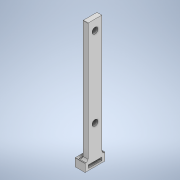
# Autodesk Inventor part: baseB
Saved by Autodesk Inventor 2021.4 (Build 254397000, 397)
## iProperties
Created: 2023-11-06
Part Number: baseB
Material: 一般
Document SubType Name: Modeling
Designer: ryusei
Density: 1 g/cm^3
Appearance: 既定
Author: ryusei
Autodesk Inventor part; units mm, degrees
ref_plane "YZ Plane" through (0, 0, 0) normal (1, 0, 0) x (0, 1, 0)
ref_plane "XZ Plane" through (0, 0, 0) normal (0, 1, 0) x (-1, 0, 0)
ref_plane "XY Plane" through (0, 0, 0) normal (0, 0, 1) x (1, 0, 0)
sketch "スケッチ1" plane through (0, 0, 0) normal (0, 1, 0) x (-1, 0, 0)
  line L0 (5, -10) -> (-5, -10)
  line L1 (-5, -10) -> (-5, 10)
  line L2 (-5, 10) -> (5, 10)
  line L3 (5, 10) -> (5, -10)
  line L4 (5, -10) -> (-5, 10) construction
  line L5 (-5, -10) -> (5, 10) construction
  point P0 (0, 0)
  dimension "d0" = 10
  dimension "d1" = 20
  constraints: 12 end point, 2 midpoint, 2 parallel, 1 horizontal, 1 perpendicular
  measures "d0" distance of L1.end L2.end
  measures "d1" distance of L0.end L1.end
extrude "押し出し1" add sketch "スケッチ1" along normal blind 6
sketch "スケッチ2" plane through (0, 0, 0) normal (0, -1, 0) x (1, 0, 0)
  line L0 (5, 10) -> (5, -10) projected
  circle A0 centre (5, 0) radius 6.75
  point P0 (0, 0)
  point P1 (5, -6.75)
  point P2 (5, 6.75)
  dimension "d4" = 13.5
  constraints: 1 centre point, 1 midpoint
  measures "d4" diameter of A0
extrude "押し出し2" cut sketch "スケッチ2" against normal blind 3 contours L0 A0 picked at (3.1483, 1.2781)
sketch "スケッチ3" plane through (0, 0, 0) normal (0, -1, 0) x (1, 0, 0)
  line L0 (-5, 10) -> (5, 10)
  line L1 (5, 10) -> (5, -10)
  line L2 (5, -10) -> (-5, -10)
  line L3 (-5, -10) -> (-5, 10)
  line L4 (-5, 10) -> (5, -10) construction
  line L5 (5, 10) -> (-5, -10) construction
  point P0 (0, 0)
  dimension "d7" = 10
  dimension "d8" = 20
  constraints: 12 end point, 2 midpoint, 2 parallel, 1 horizontal, 1 perpendicular
  measures "d7" distance of L1.end L2.end
  measures "d8" distance of L0.end L1.end
extrude "押し出し3" add sketch "スケッチ3" along normal blind 2
sketch "スケッチ4" plane through (0, 6, 0) normal (0, 1, 0) x (1, 0, 0)
  line L0 (5, 7) -> (0, 7)
  line L1 (0, 7) -> (0, -7)
  line L2 (0, -7) -> (5, -7)
  line L3 (5, -7) -> (5, 7)
  line L4 (5, -10) -> (5, 10) projected
  point P0 (0, 0)
  dimension "d11" = 5
  dimension "d12" = 14
  dimension "d13" = 5
  dimension "d14" = 7
  constraints: 8 end point, 2 parallel, 1 horizontal, 1 perpendicular
  measures "d11" distance of L2.end L1.end
  measures "d12" distance of L1.end L0.end
  measures "d13" distance between parallel lines of L4 L1
  measures "d14" distance from line of point (0, 0) L0
extrude "押し出し4" add sketch "スケッチ4" along normal blind 120
fillet "フィレット1" radius 2 3 edges at (2.5, 6, 7) (2.5, 6, -7) (0, 6, 0)
fillet "フィレット2" radius 0.2 12 edges at (-0.5858, 6.5858, -7.5858) (0, 67, -7) (-0.5858, 6.5858, 7.5858) (0, 67, 7) (2.5, 126, 7) (0, 126, 0) (2.5, 126, -7) (0, 6, -10) (-5, 6, 0) (0, 6, 10) (-5, 2, 10) (-5, 2, -10)
sketch "スケッチ5" plane through (0, 8, 6.8) normal (-1, 0, 0) x (0, 0, 1)
  line L0 (3, -2) -> (-16.6, -2) projected
  line L1 (-13.8, 117.8) -> (-13.8, 0) projected
  point P0 (-6.8, -8)
  point P1 (-6.8, 28)
  point P2 (-6.8, 108)
  dimension "d19" = 30
  dimension "d20" = 80
  dimension "d21" = 7
  dimension "d22" = 7
  measures "d19" distance from line of point (-6.8, 28) L0
  measures "d20" distance of point (-6.8, 108) point (-6.8, 28)
  measures "d21" distance from line of L1 point (-6.8, 28)
  measures "d22" distance from line of L1 point (-6.8, 108)
hole "穴1" at (0, 36, 0) at (0, 116, 0) direction (1, 0, 0) diameter 6 end through all
